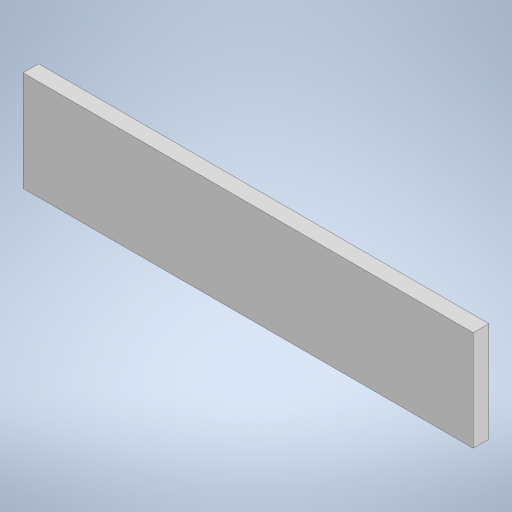
# Autodesk Inventor part: Portabateria
Saved by Autodesk Inventor 2024 (Build 280153000, 153)
## iProperties
Created: 2024-05-03
Part Number: Portabateria
Material: Generic
Document SubType Name: Modeling
Designer: samue
Density: 1 g/cm^3
Appearance: Default
Author: samue
Autodesk Inventor part; units mm, degrees
ref_plane "YZ Plane" through (0, 0, 0) normal (1, 0, 0) x (0, 1, 0)
ref_plane "XZ Plane" through (0, 0, 0) normal (0, 1, 0) x (-1, 0, 0)
ref_plane "XY Plane" through (0, 0, 0) normal (0, 0, 1) x (1, 0, 0)
sketch "Sketch1" plane through (0, 0, 0) normal (0, 1, 0) x (-1, 0, 0)
  line L0 (45, 1.5625) -> (-45, 1.5625)
  line L1 (-45, 1.5625) -> (-45, -1.5625)
  line L2 (-45, -1.5625) -> (45, -1.5625)
  line L3 (45, -1.5625) -> (45, 1.5625)
  line L4 (45, 1.5625) -> (-45, -1.5625) construction
  line L5 (-45, 1.5625) -> (45, -1.5625) construction
  point P0 (0, 0)
  dimension "d0" = 90
  dimension "d1" = 3.125
  constraints: 12 end point, 2 midpoint, 2 parallel, 1 horizontal, 1 perpendicular
  measures "d0" distance of L2.end L1.end
  measures "d1" distance of L1.end L0.end
extrude "Extrusion1" add sketch "Sketch1" along normal blind 20
body "Solid1"
